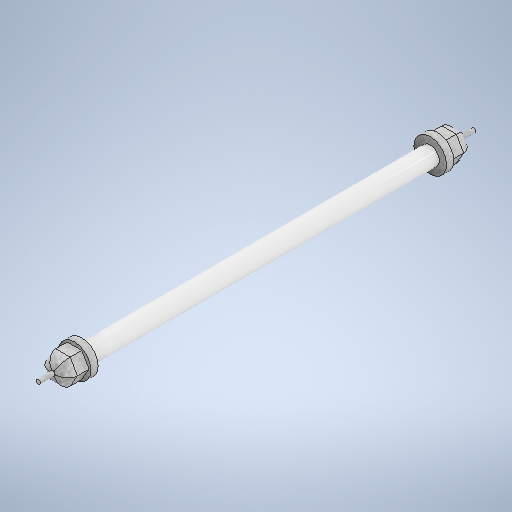
# Autodesk Inventor part: Resistencia
Saved by Autodesk Inventor 2025 (Build 290162000, 162)
## iProperties
Created: 2024-11-20
Part Number: Resistencia
Material: Generic
Document SubType Name: Sheet Metal
Designer: g.marin
Density: 1 g/cm^3
Sheet Metal Rule: Default
Appearance: Default
Author: g.marin
Autodesk Inventor part; units mm, degrees
ref_plane "YZ Plane" through (0, 0, 0) normal (1, 0, 0) x (0, 1, 0)
ref_plane "XZ Plane" through (0, 0, 0) normal (0, 1, 0) x (-1, 0, 0)
ref_plane "XY Plane" through (0, 0, 0) normal (0, 0, 1) x (1, 0, 0)
sketch "Sketch2" plane through (0, 0, 0) normal (0, 1, 0) x (-1, 0, 0)
  line L0 (0, 0) -> (6.25, 0)
  line L1 (6.25, 0) -> (6.25, -240)
  line L2 (6.25, -240) -> (0, -240)
  line L3 (0, -240) -> (0, 0)
  line L4 (0, 0) -> (11.25, 0)
  line L5 (11.25, 0) -> (11.25, 5)
  line L6 (11.25, 5) -> (0, 5)
  line L7 (0, 5) -> (0, 0)
  line L8 (0, -240) -> (11.25, -240)
  line L9 (11.25, -240) -> (11.25, -245)
  line L10 (11.25, -245) -> (0, -245)
  line L11 (0, -245) -> (0, -240)
  dimension "d15" = 6.25
  dimension "d16" = 240
  dimension "d17" = 11.25
  dimension "d18" = 5
  dimension "d19" = 5
  constraints: 24 end point, 6 parallel, 3 horizontal, 3 perpendicular, 1 point on line
  measures "d15" distance of L1.end L2.end
  measures "d16" distance of L0.end L1.end
  measures "d17" distance of L5.end L6.end
  measures "d18" distance between parallel lines of L0 L6
  measures "d19" distance between parallel lines of L10 L8
revolve "Revolution1" add sketch "Sketch2" angle 360 about axis through (0, 0, -240) along (0, 0, 1)
sketch "Sketch3" plane through (0, 0, 5) normal (0, 0, 1) x (1, 0, 0)
  line L0 (-10, -0.0006) -> (-5.0005, 8.66)
  line L1 (-5.0005, 8.66) -> (4.9995, 8.6606)
  line L2 (4.9995, 8.6606) -> (10, 0.0006)
  line L3 (10, 0.0006) -> (5.0005, -8.66)
  line L4 (5.0005, -8.66) -> (-4.9995, -8.6606)
  line L5 (-4.9995, -8.6606) -> (-10, -0.0006)
  point P0 (0, 0)
  point P1 (0, 0)
  dimension "d21" = 10
  constraints: 12 end point, 1 coincident, 13 other
  measures "d21" distance of L3.end L4.end
extrude "Extrusion1" add sketch "Sketch3" along normal blind 15
sketch "Sketch4" plane through (0, 0, -245) normal (0, 0, -1) x (-1, 0, 0)
  line L0 (-5, -8.6603) -> (-10, 0)
  line L1 (-10, 0) -> (-5, 8.6603)
  line L2 (-5, 8.6603) -> (5, 8.6603)
  line L3 (5, 8.6603) -> (10, 0)
  line L4 (10, 0) -> (5, -8.6603)
  line L5 (5, -8.6603) -> (-5, -8.6603)
  point P0 (0, 0)
  point P1 (0, 0)
  dimension "d24" = 10
  constraints: 12 end point, 1 coincident, 13 other
  measures "d24" distance of L4.end L0.start
extrude "Extrusion2" add sketch "Sketch4" along normal blind 15
fillet "Fillet1" radius 7 12 edges at (0, 8.6603, -260) (7.5, 4.3301, -260) (7.5, -4.3301, -260) (0, -8.6603, -260) (-7.5, -4.3301, -260) (-7.5, 4.3301, -260) (-7.5003, 4.3297, 20) (-0.0005, 8.6603, 20) (7.4997, 4.3306, 20) (7.5003, -4.3297, 20) (0.0005, -8.6603, 20) (-7.4997, -4.3306, 20)
sketch "Sketch5" plane through (0, 0, 20) normal (0, 0, 1) x (1, 0, 0)
  circle A0 centre (0, 0) radius 6.25 projected
  circle A1 centre (0, 0) radius 1.5
  point P0 (0, 0)
  dimension "d28" = 3
  constraints: 1 centre point, 1 coincident
  measures "d28" diameter of A1
extrude "Extrusion3" add sketch "Sketch5" along normal blind 10 contours A1
sketch "Sketch6" plane through (0, 0, -260) normal (0, 0, -1) x (-1, 0, 0)
  circle A0 centre (0, 0) radius 1.5
  dimension "d31" = 3
  constraints: 1 centre point, 1 coincident
  measures "d31" diameter of A0
extrude "Extrusion4" add sketch "Sketch6" along normal blind 10
body "Solid1"
